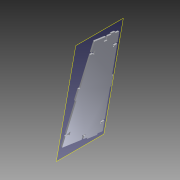
# Autodesk Inventor part: Panel_side
Saved by Autodesk Inventor 2013 (Build 170138000, 138)
## iProperties
Created: 2013-02-02
Part Number: Panel_side
Material: Aluminum 6061
Document SubType Name: Modeling
Designer: xylzlyx
Density: 1 g/cm^3
ScrewLen: 0.525 in
ScrewHoleD: 0.150 in
NutFlatsGap: 0.323 in
NutHeightGap: 0.119 in
SlotFilletRad: 0.020 in
ScrewHoleDist: 1.000 in
MetalThickness: 0.125 in
SlotWidth: 0.150 in
TabLength: 1.000 in
SlotLength: 1.050 in
SmallSlotLength: 0.425 in
SmallTabLength: 0.375 in
Author: xylzlyx
Autodesk Inventor part; units mm, degrees
ref_plane "YZ Plane" through (0, 0, 0) normal (1, 0, 0) x (0, 1, 0)
ref_plane "XZ Plane" through (0, 0, 0) normal (0, 1, 0) x (-1, 0, 0)
ref_plane "XY Plane" through (0, 0, 0) normal (0, 0, 1) x (1, 0, 0)
ref_plane "Work Plane1" through (-221.4413, -90.9255, -118.1004) normal (-0.9848078, 0.1736482, 0) x (-0.1736482, -0.9848078, 0)
sketch "Sketch1" plane through (-221.4413, -90.9255, -118.1004) normal (-0.9848078, 0.1736482, 0) x (-0.1736482, -0.9848078, 0)
  line L0 (0, 0) -> (-0.5513, 3.1268) construction
  line L1 (-0.5513, 3.1268) -> (245.7896, 46.5633) construction
  line L2 (245.7896, 46.5633) -> (246.341, 43.4366) construction
  line L3 (246.341, 43.4366) -> (0, 0) construction
  line L4 (254.4978, -57.6752) -> (251.371, -58.2265) construction
  line L5 (251.371, -58.2265) -> (233.8339, 41.2312) construction
  line L6 (233.8339, 41.2312) -> (236.9607, 41.7826) construction
  line L7 (236.9607, 41.7826) -> (254.4978, -57.6752) construction
  line L8 (12.5071, 2.2053) -> (23.1628, -58.2265) construction
  line L9 (23.1628, -58.2265) -> (20.0361, -58.7779) construction
  line L10 (20.0361, -58.7779) -> (9.3803, 1.654) construction
  line L11 (9.3803, 1.654) -> (12.5071, 2.2053) construction
  line L12 (264.2669, -61.4015) -> (10.2669, -61.4015) construction
  line L13 (10.2669, -61.4015) -> (10.2669, -58.2265) construction
  line L14 (10.2669, -58.2265) -> (264.2669, -58.2265) construction
  line L15 (264.2669, -58.2265) -> (264.2669, -61.4015) construction
  line L16 (233.8339, 41.2312) -> (251.371, -58.2265)
  line L17 (251.371, -58.2265) -> (23.1628, -58.2265)
  line L18 (23.1628, -58.2265) -> (12.5071, 2.2053)
  line L19 (12.5071, 2.2053) -> (233.8339, 41.2312)
  point P0 (-127.997, 118.1004)
  constraints: 40 end point, 4 collinear, 2 horizontal, 2 vertical, 28 other
extrude "SidePanel" add sketch "Sketch1" against normal blind 3.175
fillet "CornerFillet" radius 1 4 edges at (-263.5281, -338.7532, -176.327) (-260.4828, -321.4826, -76.8692) (-223.9001, -114.0121, -176.327) (-222.0498, -103.5182, -115.8951)
sketch "ScrewSketch" plane through (-221.4413, -90.9255, -118.1004) normal (-0.9848078, 0.1736482, 0) x (0, 0, 1)
  line L0 (-57.0529, -251.164) -> (40.2464, -234.0076) projected
  line L1 (41.0576, -232.8491) -> (2.379, -13.4919) projected
  line L2 (-61.4015, -11.2669) -> (-61.4015, -263.2669) projected
  line L3 (-58.2265, -250.1792) -> (-58.2265, -24.0019) projected
  line L4 (-61.4015, -226.6779) -> (-48.0665, -226.6779)
  line L5 (-61.4015, -222.8806) -> (-48.0665, -222.8806)
  line L6 (-61.4015, -222.8806) -> (-61.4015, -226.6779)
  line L7 (-48.0665, -226.6779) -> (-48.0665, -222.8806)
  line L8 (-61.4015, -47.5033) -> (-48.0665, -47.5033)
  line L9 (-48.0665, -47.5033) -> (-48.0665, -51.3006)
  line L10 (-48.0665, -51.3006) -> (-61.4015, -51.3006)
  line L11 (-61.4015, -51.3006) -> (-61.4015, -47.5033)
  line L12 (3.3004, -0.4335) -> (46.3897, -244.8048) projected
  line L13 (-3.5457, -38.4004) -> (9.5867, -36.0848)
  line L14 (-3.5457, -38.4004) -> (-2.8863, -42.1401)
  line L15 (-2.8863, -42.1401) -> (10.2461, -39.8245)
  line L16 (10.2461, -39.8245) -> (9.5867, -36.0848)
  line L17 (26.971, -211.4691) -> (40.1034, -209.1535)
  line L18 (26.971, -211.4691) -> (26.3116, -207.7294)
  line L19 (26.3116, -207.7294) -> (39.444, -205.4138)
  line L20 (39.444, -205.4138) -> (40.1034, -209.1535)
  line L21 (40.7978, -237.1343) -> (-56.6904, -254.3241) projected
  line L22 (0.6692, -9.5539) -> (-57.2417, -19.7652) projected
  line L23 (-48.0665, -228.875) -> (-48.0665, -220.6835)
  line L24 (-48.0665, -220.6835) -> (-51.0987, -220.6835)
  line L25 (-48.0665, -228.875) -> (-51.0987, -228.875)
  line L26 (-51.0987, -228.875) -> (-51.0987, -220.6835)
  line L27 (-48.0665, -45.3062) -> (-48.0665, -53.4977)
  line L28 (-48.0665, -53.4977) -> (-51.0987, -53.4977)
  line L29 (-51.0987, -53.4977) -> (-51.0987, -45.3062)
  line L30 (-51.0987, -45.3062) -> (-48.0665, -45.3062)
  line L31 (-2.5048, -44.3038) -> (-3.9272, -36.2367)
  line L32 (-2.5048, -44.3038) -> (0.4813, -43.7773)
  line L33 (0.4813, -43.7773) -> (-0.9412, -35.7102)
  line L34 (-0.9412, -35.7102) -> (-3.9272, -36.2367)
  line L35 (27.3525, -213.6328) -> (25.93, -205.5657)
  line L36 (25.93, -205.5657) -> (28.9161, -205.0392)
  line L37 (28.9161, -205.0392) -> (30.3385, -213.1062)
  line L38 (30.3385, -213.1062) -> (27.3525, -213.6328)
  line L39 (-6.0765, -245.3995) -> (-8.3921, -232.2671)
  line L40 (-12.1317, -232.9265) -> (-9.8161, -246.0589)
  line L41 (-8.3921, -232.2671) -> (-12.1317, -232.9265)
  line L42 (-6.0765, -245.3995) -> (-9.8161, -246.0589)
  line L43 (-14.2955, -233.308) -> (-6.2284, -231.8856)
  line L44 (-13.7689, -236.2941) -> (-14.2955, -233.308)
  line L45 (-13.7689, -236.2941) -> (-5.7019, -234.8716)
  line L46 (-5.7019, -234.8716) -> (-6.2284, -231.8856)
  line L47 (-26.4165, -14.3299) -> (-24.1009, -27.4623)
  line L48 (-24.1009, -27.4623) -> (-27.8405, -28.1217)
  line L49 (-27.8405, -28.1217) -> (-30.1561, -14.9893)
  line L50 (-30.1561, -14.9893) -> (-26.4165, -14.3299)
  line L51 (-30.0042, -28.5032) -> (-21.9371, -27.0808)
  line L52 (-21.9371, -27.0808) -> (-22.4637, -24.0947)
  line L53 (-22.4637, -24.0947) -> (-30.5307, -25.5171)
  line L54 (-30.5307, -25.5171) -> (-30.0042, -28.5032)
  line L55 (-61.4015, -224.7792) -> (-48.0665, -224.7792) construction
  line L56 (-61.4015, -49.4019) -> (-48.0665, -49.4019) construction
  line L57 (9.9164, -37.9547) -> (-3.216, -40.2702) construction
  line L58 (39.7737, -207.2836) -> (26.6413, -209.5992) construction
  point P0 (-7.9463, -245.7292)
  point P1 (-10.2619, -232.5968)
  point P2 (-28.2863, -14.6596)
  point P3 (-25.9707, -27.792)
  dimension "d7" = 13.335
  dimension "d8" = 3.7973
  dimension "d10" = 13.335
  dimension "d11" = 3.7973
  dimension "d14" = 13.335
  dimension "d17" = 3.7973
  dimension "d18" = 13.335
  dimension "d20" = 3.7973
  dimension "d21" = 8.1915
  dimension "d22" = 3.0321
  dimension "d23" = 8.1915
  dimension "d24" = 3.0321
  dimension "d25" = 8.1915
  dimension "d26" = 3.0321
  dimension "d27" = 8.1915
  dimension "d28" = 3.0321
  dimension "d29" = 13.335
  dimension "d30" = 3.7973
  dimension "d31" = 8.1915
  dimension "d32" = 3.0321
  dimension "d33" = 3.7973
  dimension "d34" = 13.335
  dimension "d35" = 8.1915
  dimension "d36" = 3.0321
  dimension "d40" = 25.4
  dimension "d41" = 25.4
  dimension "d42" = 25.4
  dimension "d43" = 25.4
  constraints: 104 end point, 39 parallel, 16 midpoint, 9 collinear, 6 perpendicular, 6 point on line
  measures "d7" distance of L4.start L4.end
  measures "d8" distance between parallel lines of L4 L5
  measures "d10" distance of L8.start L8.end
  measures "d11" distance of L10.end L8.start
  measures "d14" distance of L13.start L13.end
  measures "d17" distance between parallel lines of L13 L15
  measures "d18" distance of L17.start L17.end
  measures "d20" distance of L19.end L17.end
  measures "d21" distance of L23.start L23.end
  measures "d22" distance of L23.end L24.end
  measures "d23" distance of L27.start L27.end
  measures "d24" distance of L27.end L28.end
  measures "d25" distance of L31.start L31.end
  measures "d26" distance of L31.start L32.end
  measures "d27" distance of L35.start L35.end
  measures "d28" distance of L35.end L36.end
  measures "d29" distance of L39.start L39.end
  measures "d30" distance of L39.end L40.start
  measures "d31" distance of L43.start L43.end
  measures "d32" distance of L44.start L43.start
  measures "d33" distance of L49.end L47.start
  measures "d34" distance of L48.end L49.end
  measures "d35" distance of L51.start L51.end
  measures "d36" distance of L51.end L52.end
  measures "d40" vertical distance of L55.start L3.start
  measures "d41" vertical distance of L3.end L56.start
  measures "d42" distance from line of L1.end L57
  measures "d43" distance from line of L1.start L58
extrude "ScrewSlots" cut sketch "ScrewSketch" against normal blind 25.4 contours L40 L45 L39 L0 | L0 L39 L21 L40 | L45 L44 L43 L40 | L40 L41 L39 L45 | L39 L43 L46 L45 | L17 L37 L19 L1 | L1 L19 L12 L17 | L37 L38 L35 L17 | L17 L18 L19 L37 | L15 L33 L13 L1 | L1 L13 L12 L15 | L19 L35 L36 L37 | L33 L32 L31 L15 | L15 L14 L13 L33 | L13 L31 L34 L33 | L8 L3 L10 L2 | L8 L29 L10 L3 | L5 L3 L4 L2 | L29 L30 L27 L8 | L8 L9 L10 L29 | L5 L26 L4 L3 | L10 L27 L28 L29 | L26 L24 L23 L5 | L5 L7 L4 L26 | L4 L23 L25 L26 | L47 L53 L49 L22 | L53 L52 L51 L47 | L47 L48 L49 L53 | L49 L51 L54 L53
fillet "SlotFillets" radius 0.5 48 edges at (-261.9482, -329.7932, -124.7283) (-260.7292, -322.8803, -125.966) (-262.0627, -330.4426, -128.4679) (-260.8437, -323.5296, -129.7056) (-260.91, -323.9054, -131.8694) (-260.3915, -320.9647, -132.3959) (-260.1445, -319.5638, -124.3288) (-260.663, -322.5045, -123.8023) (-256.5077, -298.939, -88.1434) (-256.8835, -301.0698, -87.7619) (-256.9749, -301.5883, -90.748) (-255.5741, -293.6438, -92.1704) (-255.4826, -293.1253, -89.1843) (-255.8584, -295.2562, -88.8028) (-256.2928, -297.72, -81.1238) (-255.6434, -294.0372, -81.7832) (-259.6217, -316.599, -166.167) (-259.6217, -316.599, -169.1991) (-259.2402, -314.4353, -169.1991) (-259.2402, -314.4353, -176.327) (-258.5808, -310.6957, -176.327) (-258.5808, -310.6957, -169.1991) (-258.1992, -308.5319, -169.1991) (-258.1992, -308.5319, -166.167) (-229.1677, -143.8861, -166.167) (-229.1677, -143.8861, -169.1991) (-228.7862, -141.7223, -169.1991) (-228.7862, -141.7223, -176.327) (-228.1268, -137.9827, -176.327) (-228.1268, -137.9827, -169.1991) (-227.7453, -135.819, -169.1991) (-227.7453, -135.819, -166.167) (-224.8275, -119.2713, -148.1046) (-224.5805, -117.8705, -140.0376) (-224.062, -114.9298, -140.5641) (-224.1282, -115.3055, -142.7278) (-224.2427, -115.9549, -146.4674) (-224.309, -116.3306, -148.6312) (-223.0238, -109.0419, -147.7052) (-222.9093, -108.3926, -143.9656) (-226.1704, -126.8873, -122.0277) (-227.4798, -134.3133, -117.6192) (-227.5712, -134.8318, -120.6052) (-226.079, -126.3688, -119.0416) (-226.2398, -127.2807, -111.6405) (-226.8891, -130.9635, -110.9811) (-226.4547, -128.4997, -118.6601) (-227.1041, -132.1825, -118.0007)
sketch "TopTabSketch" plane through (-260.0573, -309.9276, -176.327) normal (0, 0, -1) x (-0.9848078, 0.1736482, 0)
  line L0 (0, 72.59) -> (-3.175, 72.59)
  line L1 (-3.175, 72.59) -> (-3.175, 97.99)
  line L2 (-3.175, 97.99) -> (0, 97.99)
  line L3 (0, 97.99) -> (0, 72.59)
  line L4 (-2.9925, 71.955) -> (-0.1825, 71.955) projected
  line L5 (0.3175, 72.455) -> (0.3175, 98.125) projected
  point P0 (-1.5875, 85.29)
  point P1 (0, 85.29)
  point P2 (-1.5875, 72.59)
  point P3 (0.3175, 85.29)
  point P4 (-1.5875, 71.955)
  point P5 (-3.175, -27.7987)
  dimension "d44" = 25.4
  constraints: 8 end point, 4 midpoint, 3 vertical alignment, 2 horizontal alignment, 2 parallel, 1 horizontal, 1 perpendicular
  measures "d44" distance of L0.end L1.end
extrude "TopTab" add sketch "TopTabSketch" along normal blind 3.175
fillet "TopTabFillet" radius 0.5 4 edges at (-245.8888, -238.7161, -179.502) (-245.8888, -238.7161, -176.327) (-241.4782, -213.7019, -179.502) (-241.4782, -213.7019, -176.327)
sketch "BottomTabSketch" plane through (-257.1213, -293.2766, -81.87) normal (0.0301537, 0.1710101, 0.9848078) x (0.9848078, -0.1736482, 0)
  line L0 (3.175, 96.2719) -> (0, 96.2719)
  line L1 (0, 96.2719) -> (0, 70.8719)
  line L2 (0, 70.8719) -> (3.175, 70.8719)
  line L3 (3.175, 70.8719) -> (3.175, 96.2719)
  line L4 (2.9925, 96.9069) -> (0.1825, 96.9069) projected
  line L5 (-0.3175, 96.4069) -> (-0.3175, 70.7369) projected
  point P0 (3.175, 167.1439)
  point P1 (202.2881, 314.187)
  point P2 (1.5875, 96.2719)
  point P3 (1.5875, 96.9069)
  point P4 (0, 83.5719)
  point P5 (-0.3175, 83.5719)
  dimension "d50" = 25.4
  constraints: 8 end point, 4 midpoint, 2 parallel, 2 vertical alignment, 1 horizontal, 1 horizontal alignment, 1 perpendicular
  measures "d50" distance of L2.end L0.start
extrude "BottomTab" add sketch "BottomTabSketch" along normal blind 3.175
fillet "BottomTabFillet" radius 0.5 4 edges at (-239.0945, -200.1833, -98.5875) (-238.9987, -199.6404, -95.4607) (-243.3424, -224.2745, -91.0501) (-243.4381, -224.8174, -94.1768)
sketch "BackTabSketch" plane through (-265.0555, -338.2738, -175.1533) normal (-0.1710101, -0.9698463, 0.1736482) x (0.9848078, -0.1736482, 0)
  line L0 (0, 11.3563) -> (3.175, 11.3563)
  line L1 (3.175, 11.3563) -> (3.175, 36.7563)
  line L2 (3.175, 36.7563) -> (0, 36.7563)
  line L3 (0, 36.7563) -> (0, 11.3563)
  line L4 (2.9925, 37.3913) -> (0.1825, 37.3913) projected
  line L5 (-0.3175, 36.8913) -> (-0.3175, 11.2213) projected
  point P0 (0, 0)
  point P1 (202.2881, 238.333)
  point P2 (3.175, 24.0563)
  point P3 (-0.3175, 24.0563)
  point P4 (1.5875, 36.7563)
  point P5 (1.5875, 37.3913)
  dimension "d56" = 25.4
  constraints: 8 end point, 4 midpoint, 2 parallel, 2 vertical alignment, 1 horizontal, 1 horizontal alignment, 1 perpendicular
  measures "d56" distance of L0.end L1.end
extrude "BackTab" add sketch "BackTabSketch" along normal blind 3.175
fillet "BackTabFillet" radius 0.5 4 edges at (-262.3838, -332.2637, -138.9555) (-262.9268, -335.343, -138.4042) (-263.6927, -339.6867, -163.4183) (-263.1497, -336.6074, -163.9696)
sketch "FrontTabSketch" plane through (-225.4382, -113.5929, -175.5006) normal (0.1710101, 0.9698463, -0.1736482) x (0.9848078, -0.1736482, 0)
  line L0 (3.175, -10.1593) -> (0, -10.1593)
  line L1 (0, -10.1593) -> (0, -19.6843)
  line L2 (0, -19.6843) -> (3.175, -19.6843)
  line L3 (3.175, -19.6843) -> (3.175, -10.1593)
  line L4 (2.9925, -9.5243) -> (0.1825, -9.5243) projected
  line L5 (-0.3175, -10.0243) -> (-0.3175, -19.8193) projected
  point P0 (3.175, 0)
  point P1 (202.2881, -199.0577)
  point P2 (1.5875, -9.5243)
  point P3 (1.5875, -10.1593)
  point P4 (-0.3175, -14.9218)
  point P5 (0, -14.9218)
  dimension "d61" = 9.525
  constraints: 8 end point, 4 midpoint, 2 parallel, 2 vertical alignment, 1 horizontal, 1 horizontal alignment, 1 perpendicular
  measures "d61" distance of L2.end L0.start
extrude "FrontTab" add sketch "FrontTabSketch" along normal blind 3.175
fillet "FrontTabFillet" radius 0.5 4 edges at (-223.5685, -112.1312, -165.4957) (-223.0255, -109.052, -166.047) (-222.7383, -107.4231, -156.6667) (-223.2813, -110.5023, -156.1154)
equation "\"d7\" = ScrewLen"
equation "\"d8\" = ScrewHoleD"
equation "\"d10\" = ScrewLen"
equation "\"d11\" = ScrewHoleD"
equation "\"d14\" = ScrewLen"
equation "\"d17\" = ScrewHoleD"
equation "\"d18\" = ScrewLen"
equation "\"d20\" = ScrewHoleD"
equation "\"d21\" = NutFlatsGap"
equation "\"d22\" = NutHeightGap"
equation "\"d23\" = NutFlatsGap"
equation "\"d24\" = NutHeightGap"
equation "\"d25\" = NutFlatsGap"
equation "\"d26\" = NutHeightGap"
equation "\"d27\" = NutFlatsGap"
equation "\"d28\" = NutHeightGap"
equation "\"d29\" = ScrewLen"
equation "\"d30\" = ScrewHoleD"
equation "\"d31\" = NutFlatsGap"
equation "\"d32\" = NutHeightGap"
equation "\"d33\" = ScrewHoleD"
equation "\"d34\" = ScrewLen"
equation "\"d35\" = NutFlatsGap"
equation "\"d36\" = NutHeightGap"
equation "\"ScrewLen\" = 13.335"
equation "\"ScrewHoleD\" = 3.7973"
equation "\"NutFlatsGap\" = 8.1915"
equation "\"NutHeightGap\" = 3.03212"
equation "\"SlotFilletRad\" = 0.5"
equation "\"ScrewHoleDist\" = 25.4"
equation "\"MetalThickness\" = 3.175"
equation "\"SlotWidth\" = 3.81"
equation "\"TabLength\" = 25.4"
equation "\"SlotLength\" = 26.67"
equation "\"SmallSlotLength\" = 10.795"
equation "\"SmallTabLength\" = 9.525"
body "Solid1"
